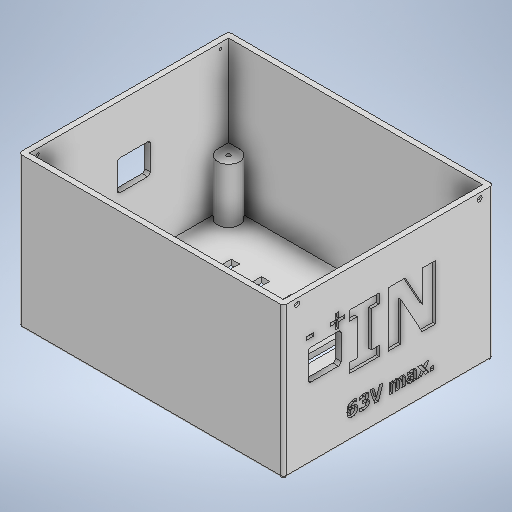
# Autodesk Inventor part: Kondensatorbox
Saved by Autodesk Inventor 2025 (Build 290162010, 162A)
## iProperties
Created: 2024-10-11
Part Number: Kondensatorbox
Material: Generisch
Document SubType Name: Modeling
Designer: max-h
Density: 1 g/cm^3
Appearance: Vorgabe
Author: max-h
Autodesk Inventor part; units mm, degrees
ref_plane "YZ Plane" through (0, 0, 0) normal (1, 0, 0) x (0, 1, 0)
ref_plane "XZ Plane" through (0, 0, 0) normal (0, 1, 0) x (-1, 0, 0)
ref_plane "XY Plane" through (0, 0, 0) normal (0, 0, 1) x (1, 0, 0)
sketch "Skizze1" plane through (0, 0, 0) normal (0, 1, 0) x (-1, 0, 0)
  line L0 (90.5, 0) -> (0, 0) construction
  line L1 (0, 0) -> (0, -70.5) construction
  line L2 (0, -70.5) -> (90.5, -70.5) construction
  line L3 (90.5, -70.5) -> (90.5, 0) construction
  line L4 (93.5, 3) -> (-3, 3)
  line L5 (-3, 3) -> (-3, -73.5)
  line L6 (-3, -73.5) -> (93.5, -73.5)
  line L7 (93.5, -73.5) -> (93.5, 3)
  dimension "d0" = 70.5
  dimension "d1" = 90.5
  dimension "d2" = 3
  dimension "d3" = 3
  dimension "d4" = 3
  dimension "d5" = 3
  constraints: 16 end point, 4 parallel, 2 horizontal, 2 perpendicular, 1 coincident
  measures "d0" distance of L2.end L0.start
  measures "d1" distance of L1.end L2.end
  measures "d2" distance between parallel lines of L7 L3
  measures "d3" distance between parallel lines of L4 L0
  measures "d4" distance between parallel lines of L5 L1
  measures "d5" distance between parallel lines of L6 L2
extrude "Extrusion1" add sketch "Skizze1" along normal blind 55
shell "Wandung1" thickness 2 removed faces 1 at (-29.1667, 55, -22.5)
sketch "Skizze4" plane through (1, 55, -71.5) normal (-1, 0, 0) x (0, 0, 1)
  line L0 (65.5, -29) -> (53.5, -29)
  line L1 (53.5, -29) -> (53.5, -18)
  line L2 (53.5, -18) -> (65.5, -18)
  line L3 (65.5, -18) -> (65.5, -29)
  line L4 (72.5, -53) -> (72.5, 0) projected
  line L5 (72.5, -53) -> (0, -53) projected
  point P0 (71.5, -55)
  dimension "d26" = 7
  dimension "d27" = 12
  dimension "d29" = 11
  dimension "d65" = 24
  constraints: 8 end point, 2 parallel, 1 horizontal, 1 perpendicular
  measures "d26" distance between parallel lines of L4 L3
  measures "d27" distance of L0.start L0.end
  measures "d29" distance of L2.end L0.start
  measures "d65" distance between parallel lines of L5 L0
extrude "Extrusion4" cut sketch "Skizze4" against normal blind 4
sketch "Skizze5" plane through (-91.5, 55, 1) normal (1, 0, 0) x (0, 0, -1)
  line L0 (32, -18) -> (44, -18)
  line L1 (44, -18) -> (44, -29)
  line L2 (44, -29) -> (32, -29)
  line L3 (32, -29) -> (32, -18)
  line L4 (19, -18) -> (19, -29) projected
  line L5 (7, -18) -> (19, -18) projected
  line L6 (0, -53) -> (0, 0) projected
  line L7 (72.5, -53) -> (0, -53) projected
  point P0 (1, -55)
  dimension "d33" = 32
  dimension "d66" = 24
  constraints: 8 end point, 2 equal length, 2 parallel, 1 horizontal, 1 perpendicular
  measures "d33" distance between parallel lines of L6 L3
  measures "d66" distance between parallel lines of L7 L2
extrude "Extrusion5" cut sketch "Skizze5" against normal blind 4
fillet "Rundung1" radius 1 16 edges at (-92.5, 26, -43) (-92.5, 26, -31) (-92.5, 37, -31) (-92.5, 37, -43) (2, 26, -6) (2, 26, -18) (2, 37, -18) (2, 37, -6) (-45.25, 0, 3) (3, 0, -35.25) (-45.25, 0, -73.5) (-93.5, 0, -35.25) (3, 27.5, -73.5) (-93.5, 27.5, -73.5) (3, 27.5, 3) (-93.5, 27.5, 3)
sketch "Skizze6" plane through (3, 0, 3) normal (1, 0, 0) x (0, 0, -1)
  circle A0 centre (5, 53) radius 0.5
  circle A1 centre (71.5, 53) radius 0.5
  line L0 (5, 53) -> (71.5, 53) construction
  line L1 (1, 55) -> (75.5, 55) construction
  line L2 (0, 55) -> (0, 1) projected
  line L3 (76.5, 1) -> (76.5, 55) projected
  point P0 (3, 0)
  dimension "d40" = 2
  dimension "d43" = 1
  dimension "d46" = 5
  dimension "d47" = 5
  constraints: 2 centre point, 2 end point, 1 coincident, 1 equal radius, 1 horizontal
  measures "d40" distance between parallel lines of L1 L0
  measures "d43" diameter of A1
  measures "d46" distance from line of L2 L0.start
  measures "d47" distance from line of L3 A1.centre
extrude "Extrusion6" cut sketch "Skizze6" against normal through all
chamfer "Fasen2" distance 0.4 angle 45 4 edges at (3, 53, -1.5) (3, 53, -68) (-93.5, 53, -68) (-93.5, 53, -1.5)
sketch "Skizze10" plane through (-91.5, 2, -71.5) normal (0, 1, 0) x (1, 0, 0)
  arc A0 (92.5, -68.5) -> (88.5, -72.5) centre (88.5, -68.5) ccw
  line L0 (0, -72.5) -> (92.5, -72.5) projected
  line L1 (92.5, -72.5) -> (92.5, 0) projected
  arc A1 (88.5, 0) -> (92.5, -4) centre (88.5, -4) ccw
  arc A2 (0, -4) -> (4, 0) centre (4, -4) ccw
  arc A3 (4, -72.5) -> (0, -68.5) centre (4, -68.5) ccw
  line L2 (0, 0) -> (0, -72.5) projected
  line L3 (92.5, 0) -> (0, 0) projected
  point P0 (91.5, -71.5)
  dimension "d67" = 4
  dimension "d68" = 4
  dimension "d69" = 4
  dimension "d70" = 4
  dimension "d71" = 4
  dimension "d72" = 4
  dimension "d73" = 4
  dimension "d74" = 4
  dimension "d75" = 8
  constraints: 8 point on circle, 8 point on line, 4 centre point, 3 equal radius
  measures "d67" distance from line of L0 A0.centre
  measures "d68" distance from line of L1 A0.centre
  measures "d69" distance from line of L0 A3.centre
  measures "d70" distance from line of L2 A3.centre
  measures "d71" distance from line of L2 A2.centre
  measures "d72" distance from line of L3 A2.centre
  measures "d73" distance from line of L3 A1.centre
  measures "d74" distance from line of L1 A1.centre
  measures "d75" diameter of A0
extrude "Extrusion10" add sketch "Skizze10" along normal blind 20 contours L1 L0 A0 | A1 L3 L1 | L0 L2 A3 | A2 L2 L3
sketch "Skizze11" plane through (-91.5, 22, -71.5) normal (0, 1, 0) x (1, 0, 0)
  arc A0 (92.5, -68.5) -> (88.5, -72.5) centre (88.5, -68.5) ccw projected
  arc A1 (4, -72.5) -> (0, -68.5) centre (4, -68.5) ccw projected
  line L0 (0, -4) -> (0, 0) projected
  arc A2 (0, -4) -> (4, 0) centre (4, -4) ccw projected
  line L1 (0, 0) -> (4, 0) projected
  arc A3 (88.5, 0) -> (92.5, -4) centre (88.5, -4) ccw projected
  circle A4 centre (88.5, -4) radius 0.75
  circle A5 centre (88.5, -68.5) radius 0.75
  circle A6 centre (4, -68.5) radius 0.75
  circle A7 centre (4, -4) radius 0.75
  point P0 (91.5, -71.5)
  dimension "d78" = 1.5
  constraints: 4 centre point, 4 coincident, 3 equal radius
  measures "d78" diameter of A5
extrude "Extrusion11" cut sketch "Skizze11" against normal blind 10 contours A4 | A5 | A6 | A7
sketch "Skizze12" plane through (-87.5, 2, -71.5) normal (0, 1, 0) x (1, 0, 0)
  line L0 (71.25, -56.25) -> (68.25, -56.25)
  line L1 (68.25, -56.25) -> (68.25, -16.25)
  line L2 (68.25, -16.25) -> (71.25, -16.25)
  line L3 (71.25, -16.25) -> (71.25, -56.25)
  line L4 (60.25, -56.25) -> (57.25, -56.25)
  line L5 (57.25, -56.25) -> (57.25, -16.25)
  line L6 (57.25, -16.25) -> (60.25, -16.25)
  line L7 (60.25, -16.25) -> (60.25, -56.25)
  line L8 (49.25, -56.25) -> (46.25, -56.25)
  line L9 (46.25, -56.25) -> (46.25, -16.25)
  line L10 (46.25, -16.25) -> (49.25, -16.25)
  line L11 (49.25, -16.25) -> (49.25, -56.25)
  line L12 (38.25, -56.25) -> (35.25, -56.25)
  line L13 (35.25, -56.25) -> (35.25, -16.25)
  line L14 (35.25, -16.25) -> (38.25, -16.25)
  line L15 (38.25, -16.25) -> (38.25, -56.25)
  line L16 (27.25, -56.25) -> (24.25, -56.25)
  line L17 (24.25, -56.25) -> (24.25, -16.25)
  line L18 (24.25, -16.25) -> (27.25, -16.25)
  line L19 (27.25, -16.25) -> (27.25, -56.25)
  line L20 (16.25, -56.25) -> (13.25, -56.25)
  line L21 (13.25, -56.25) -> (13.25, -16.25)
  line L22 (13.25, -16.25) -> (16.25, -16.25)
  line L23 (16.25, -16.25) -> (16.25, -56.25)
  line L24 (-4, -4) -> (-4, -68.5) projected
  line L25 (0, -72.5) -> (84.5, -72.5) projected
  point P0 (87.5, -71.5)
  point P1 (57.25, -36.25)
  point P2 (27.25, -36.25)
  point P3 (35.25, -36.25)
  dimension "d81" = 8
  dimension "d82" = 8
  dimension "d83" = 8
  dimension "d84" = 8
  dimension "d85" = 8
  dimension "d86" = 3
  dimension "d87" = 40
  dimension "d88" = 17.25
  dimension "d89" = 16.25
  constraints: 48 end point, 12 parallel, 9 equal length, 6 horizontal, 6 perpendicular, 4 point on line, 3 midpoint, 2 collinear
  measures "d81" distance between parallel lines of L7 L1
  measures "d82" distance from line of L11 point (57.25, -36.25)
  measures "d83" distance between parallel lines of L15 L9
  measures "d84" distance of point (27.25, -36.25) point (35.25, -36.25)
  measures "d85" distance between parallel lines of L23 L17
  measures "d86" distance of L1.end L2.end
  measures "d87" distance of L2.end L0.start
  measures "d88" distance between parallel lines of L24 L21
  measures "d89" distance between parallel lines of L25 L0
extrude "Extrusion12" cut sketch "Skizze12" against normal blind 55
sketch "Skizze13" plane through (3, 1, -72.5) normal (1, 0, 0) x (0, 0, -1)
  line L0 (-52.6804, 40.6521) -> (-18.8731, 40.6521) construction
  line L1 (-18.8731, 40.6521) -> (-18.8731, 5.4097) construction
  line L2 (-18.8731, 5.4097) -> (-52.6804, 5.4097) construction
  line L3 (-52.6804, 5.4097) -> (-52.6804, 40.6521) construction
  line L4 (-40.6545, 20.6521) -> (-51.4162, 20.6521)
  line L5 (-51.4162, 20.6521) -> (-51.4162, 24.1367)
  line L6 (-51.4162, 24.1367) -> (-48.5475, 24.1367)
  line L7 (-48.5475, 24.1367) -> (-48.5475, 37.1675)
  line L8 (-48.5475, 37.1675) -> (-51.4162, 37.1675)
  line L9 (-51.4162, 37.1675) -> (-51.4162, 40.6521)
  line L10 (-51.4162, 40.6521) -> (-40.6545, 40.6521)
  line L11 (-40.6545, 40.6521) -> (-40.6545, 37.1675)
  line L12 (-40.6545, 37.1675) -> (-43.5232, 37.1675)
  line L13 (-43.5232, 37.1675) -> (-43.5232, 24.1367)
  line L14 (-43.5232, 24.1367) -> (-40.6545, 24.1367)
  line L15 (-40.6545, 24.1367) -> (-40.6545, 20.6521)
  line L16 (-20.1844, 20.6521) -> (-25.0143, 20.6521)
  line L17 (-25.0143, 20.6521) -> (-32.729, 34.5905)
  line L18 (-32.729, 34.5905) -> (-32.729, 20.6521)
  line L19 (-32.729, 20.6521) -> (-37.3157, 20.6521)
  line L20 (-37.3157, 20.6521) -> (-37.3157, 40.6521)
  line L21 (-37.3157, 40.6521) -> (-31.1569, 40.6521)
  line L22 (-31.1569, 40.6521) -> (-24.7711, 29.1934)
  line L23 (-24.7711, 29.1934) -> (-24.7711, 40.6521)
  line L24 (-24.7711, 40.6521) -> (-20.1844, 40.6521)
  line L25 (-20.1844, 40.6521) -> (-20.1844, 20.6521)
  spline S0 degree 2 poles (-48.5272, 8.3331) (-48.5272, 7.543) (-49.528, 6.526) (-50.4032, 6.526) knots 0 0 0 1 2 2 2
  spline S1 degree 2 poles (-50.4032, 6.526) (-50.8408, 6.526) (-51.5256, 6.7772) (-51.7647, 7.0243) knots 0 0 0 1 2 2 2
  spline S2 degree 2 poles (-51.7647, 7.0243) (-52.0483, 7.312) (-52.3522, 8.2237) (-52.3522, 8.8598) knots 0 0 0 1 2 2 2
  spline S3 degree 2 poles (-52.3522, 8.8598) (-52.3522, 9.5162) (-52.0686, 10.5373) (-51.7485, 10.9303) knots 0 0 0 1 2 2 2
  spline S4 degree 2 poles (-51.7485, 10.9303) (-51.4446, 11.3031) (-50.4559, 11.7245) (-49.7792, 11.7245) knots 0 0 0 1 2 2 2
  spline S5 degree 2 poles (-49.7792, 11.7245) (-49.5321, 11.7245) (-49.0378, 11.6597) (-48.9486, 11.6394) knots 0 0 0 1 2 2 2
  line L26 (-48.9486, 11.6394) -> (-48.9486, 10.6589)
  line L27 (-48.9486, 10.6589) -> (-49.0378, 10.6589)
  spline S6 degree 2 poles (-49.0378, 10.6589) (-49.1269, 10.7034) (-49.5321, 10.8128) (-49.7914, 10.8128) knots 0 0 0 1 2 2 2
  spline S7 degree 2 poles (-49.7914, 10.8128) (-50.3789, 10.8128) (-51.0191, 10.1929) (-51.0961, 9.6175) knots 0 0 0 1 2 2 2
  spline S8 degree 2 poles (-51.0961, 9.6175) (-50.8489, 9.7755) (-50.3425, 9.9619) (-50.0224, 9.9619) knots 0 0 0 1 2 2 2
  spline S9 degree 2 poles (-50.0224, 9.9619) (-49.7509, 9.9619) (-49.2768, 9.8161) (-49.0945, 9.6783) knots 0 0 0 1 2 2 2
  spline S10 degree 2 poles (-49.0945, 9.6783) (-48.8352, 9.4798) (-48.5272, 8.8355) (-48.5272, 8.3331) knots 0 0 0 1 2 2 2
  spline S11 degree 2 poles (-49.9899, 7.5794) (-49.8927, 7.701) (-49.7874, 7.9846) (-49.7874, 8.2723) knots 0 0 0 1 2 2 2
  spline S12 degree 2 poles (-49.7874, 8.2723) (-49.7874, 8.5154) (-49.9089, 8.8315) (-50.0183, 8.9247) knots 0 0 0 1 2 2 2
  spline S13 degree 2 poles (-50.0183, 8.9247) (-50.1318, 9.0219) (-50.4113, 9.0908) (-50.5694, 9.0908) knots 0 0 0 1 2 2 2
  spline S14 degree 2 poles (-50.5694, 9.0908) (-50.7031, 9.0908) (-50.9786, 9.0219) (-51.1002, 8.9733) knots 0 0 0 1 2 2 2
  spline S15 degree 2 poles (-51.1002, 8.9733) (-51.1002, 8.9409) (-51.1083, 8.7869) (-51.1083, 8.6694) knots 0 0 0 1 2 2 2
  spline S16 degree 2 poles (-51.1083, 8.6694) (-51.1083, 8.2358) (-50.9583, 7.7132) (-50.8408, 7.5794) knots 0 0 0 1 2 2 2
  spline S17 degree 2 poles (-50.8408, 7.5794) (-50.7557, 7.47) (-50.5288, 7.3768) (-50.4073, 7.3768) knots 0 0 0 1 2 2 2
  spline S18 degree 2 poles (-50.4073, 7.3768) (-50.306, 7.3768) (-50.071, 7.4781) (-49.9899, 7.5794) knots 0 0 0 1 2 2 2
  spline S19 degree 2 poles (-44.2444, 8.1467) (-44.2444, 7.778) (-44.5159, 7.1743) (-44.7792, 6.9636) knots 0 0 0 1 2 2 2
  spline S20 degree 2 poles (-44.7792, 6.9636) (-45.0426, 6.7529) (-45.7598, 6.526) (-46.2744, 6.526) knots 0 0 0 1 2 2 2
  spline S21 degree 2 poles (-46.2744, 6.526) (-46.8579, 6.526) (-47.6925, 6.7204) (-47.9559, 6.842) knots 0 0 0 1 2 2 2
  line L28 (-47.9559, 6.842) -> (-47.9559, 7.9279)
  line L29 (-47.9559, 7.9279) -> (-47.8344, 7.9279)
  spline S22 degree 2 poles (-47.8344, 7.9279) (-47.5588, 7.7537) (-46.8173, 7.4944) (-46.5094, 7.4944) knots 0 0 0 1 2 2 2
  spline S23 degree 2 poles (-46.5094, 7.4944) (-46.3271, 7.4944) (-45.9016, 7.5592) (-45.7557, 7.6645) knots 0 0 0 1 2 2 2
  spline S24 degree 2 poles (-45.7557, 7.6645) (-45.6423, 7.7496) (-45.5045, 7.9968) (-45.5045, 8.2196) knots 0 0 0 1 2 2 2
  spline S25 degree 2 poles (-45.5045, 8.2196) (-45.5045, 8.4425) (-45.699, 8.6815) (-45.8611, 8.7383) knots 0 0 0 1 2 2 2
  spline S26 degree 2 poles (-45.8611, 8.7383) (-46.0232, 8.795) (-46.4729, 8.8072) (-46.6472, 8.8072) knots 0 0 0 1 2 2 2
  line L30 (-46.6472, 8.8072) -> (-46.8619, 8.8072)
  line L31 (-46.8619, 8.8072) -> (-46.8619, 9.6864)
  line L32 (-46.8619, 9.6864) -> (-46.6634, 9.6864)
  spline S27 degree 2 poles (-46.6634, 9.6864) (-46.4365, 9.6864) (-46.0515, 9.7269) (-45.9178, 9.7877) knots 0 0 0 1 2 2 2
  spline S28 degree 2 poles (-45.9178, 9.7877) (-45.7841, 9.8525) (-45.6342, 10.0794) (-45.6342, 10.2739) knots 0 0 0 1 2 2 2
  spline S29 degree 2 poles (-45.6342, 10.2739) (-45.6342, 10.4279) (-45.776, 10.6183) (-45.8773, 10.671) knots 0 0 0 1 2 2 2
  spline S30 degree 2 poles (-45.8773, 10.671) (-45.9989, 10.7318) (-46.323, 10.7723) (-46.4365, 10.7723) knots 0 0 0 1 2 2 2
  spline S31 degree 2 poles (-46.4365, 10.7723) (-46.6188, 10.7723) (-47.0037, 10.6872) (-47.182, 10.6183) knots 0 0 0 1 2 2 2
  spline S32 degree 2 poles (-47.182, 10.6183) (-47.3238, 10.5657) (-47.6318, 10.3955) (-47.7047, 10.3509) knots 0 0 0 1 2 2 2
  line L33 (-47.7047, 10.3509) -> (-47.81, 10.3509)
  line L34 (-47.81, 10.3509) -> (-47.81, 11.4206)
  spline S33 degree 2 poles (-47.81, 11.4206) (-47.5507, 11.53) (-46.6755, 11.7367) (-46.2177, 11.7367) knots 0 0 0 1 2 2 2
  spline S34 degree 2 poles (-46.2177, 11.7367) (-45.772, 11.7367) (-45.1156, 11.5827) (-44.8846, 11.4328) knots 0 0 0 1 2 2 2
  spline S35 degree 2 poles (-44.8846, 11.4328) (-44.6293, 11.2747) (-44.3741, 10.7885) (-44.3741, 10.4846) knots 0 0 0 1 2 2 2
  spline S36 degree 2 poles (-44.3741, 10.4846) (-44.3741, 10.0551) (-44.8684, 9.4149) (-45.2736, 9.3217) knots 0 0 0 1 2 2 2
  line L35 (-45.2736, 9.3217) -> (-45.2736, 9.2731)
  spline S37 degree 2 poles (-45.2736, 9.2731) (-45.0953, 9.2488) (-44.7549, 9.1191) (-44.5929, 8.9733) knots 0 0 0 1 2 2 2
  spline S38 degree 2 poles (-44.5929, 8.9733) (-44.4429, 8.8436) (-44.2444, 8.4303) (-44.2444, 8.1467) knots 0 0 0 1 2 2 2
  line L36 (-39.2282, 11.6313) -> (-40.9462, 6.6313)
  line L37 (-40.9462, 6.6313) -> (-42.2549, 6.6313)
  line L38 (-42.2549, 6.6313) -> (-43.9729, 11.6313)
  line L39 (-43.9729, 11.6313) -> (-42.6723, 11.6313)
  line L40 (-42.6723, 11.6313) -> (-41.5823, 8.2399)
  line L41 (-41.5823, 8.2399) -> (-40.4964, 11.6313)
  line L42 (-40.4964, 11.6313) -> (-39.2282, 11.6313)
  line L43 (-32.3157, 6.6313) -> (-32.3157, 8.5154)
  spline S39 degree 2 poles (-32.3157, 8.5154) (-32.3157, 8.795) (-32.336, 9.1759) (-32.3846, 9.2974) knots 0 0 0 1 2 2 2
  spline S40 degree 2 poles (-32.3846, 9.2974) (-32.4373, 9.419) (-32.648, 9.5284) (-32.8384, 9.5284) knots 0 0 0 1 2 2 2
  spline S41 degree 2 poles (-32.8384, 9.5284) (-32.9721, 9.5284) (-33.2314, 9.4109) (-33.3854, 9.3015) knots 0 0 0 1 2 2 2
  line L44 (-33.3854, 9.3015) -> (-33.3854, 6.6313)
  line L45 (-33.3854, 6.6313) -> (-34.5686, 6.6313)
  line L46 (-34.5686, 6.6313) -> (-34.5686, 8.5154)
  spline S42 degree 2 poles (-34.5686, 8.5154) (-34.5686, 8.7909) (-34.5929, 9.1759) (-34.6415, 9.2974) knots 0 0 0 1 2 2 2
  spline S43 degree 2 poles (-34.6415, 9.2974) (-34.6942, 9.419) (-34.9049, 9.5284) (-35.0953, 9.5284) knots 0 0 0 1 2 2 2
  spline S44 degree 2 poles (-35.0953, 9.5284) (-35.2371, 9.5284) (-35.5167, 9.3947) (-35.6463, 9.3015) knots 0 0 0 1 2 2 2
  line L47 (-35.6463, 9.3015) -> (-35.6463, 6.6313)
  line L48 (-35.6463, 6.6313) -> (-36.8214, 6.6313)
  line L49 (-36.8214, 6.6313) -> (-36.8214, 10.4036)
  line L50 (-36.8214, 10.4036) -> (-35.6463, 10.4036)
  line L51 (-35.6463, 10.4036) -> (-35.6463, 9.9862)
  spline S45 degree 2 poles (-35.6463, 9.9862) (-35.3587, 10.2294) (-34.8441, 10.5049) (-34.524, 10.5049) knots 0 0 0 1 2 2 2
  spline S46 degree 2 poles (-34.524, 10.5049) (-34.1796, 10.5049) (-33.6528, 10.1767) (-33.5151, 9.8485) knots 0 0 0 1 2 2 2
  spline S47 degree 2 poles (-33.5151, 9.8485) (-33.1788, 10.1645) (-32.5791, 10.5049) (-32.2711, 10.5049) knots 0 0 0 1 2 2 2
  spline S48 degree 2 poles (-32.2711, 10.5049) (-32.0078, 10.5049) (-31.5904, 10.3388) (-31.4486, 10.1686) knots 0 0 0 1 2 2 2
  spline S49 degree 2 poles (-31.4486, 10.1686) (-31.2906, 9.9862) (-31.1326, 9.4879) (-31.1326, 9.0867) knots 0 0 0 1 2 2 2
  line L52 (-31.1326, 9.0867) -> (-31.1326, 6.6313)
  line L53 (-31.1326, 6.6313) -> (-32.3157, 6.6313)
  spline S50 degree 2 poles (-28.1828, 7.0324) (-28.3044, 6.9311) (-28.4948, 6.7691) (-28.6569, 6.688) knots 0 0 0 1 2 2 2
  spline S51 degree 2 poles (-28.6569, 6.688) (-28.8149, 6.611) (-29.1147, 6.53) (-29.3822, 6.53) knots 0 0 0 1 2 2 2
  spline S52 degree 2 poles (-29.3822, 6.53) (-29.8846, 6.53) (-30.5451, 7.2026) (-30.5451, 7.7132) knots 0 0 0 1 2 2 2
  spline S53 degree 2 poles (-30.5451, 7.7132) (-30.5451, 8.1305) (-30.2087, 8.6491) (-29.8927, 8.7991) knots 0 0 0 1 2 2 2
  spline S54 degree 2 poles (-29.8927, 8.7991) (-29.5726, 8.953) (-28.6852, 9.0746) (-28.1747, 9.107) knots 0 0 0 1 2 2 2
  line L54 (-28.1747, 9.107) -> (-28.1747, 9.1273)
  spline S55 degree 2 poles (-28.1747, 9.1273) (-28.1747, 9.4392) (-28.6366, 9.6783) (-29.0985, 9.6783) knots 0 0 0 1 2 2 2
  spline S56 degree 2 poles (-29.0985, 9.6783) (-29.3052, 9.6783) (-29.8643, 9.5284) (-30.1277, 9.4109) knots 0 0 0 1 2 2 2
  line L55 (-30.1277, 9.4109) -> (-30.229, 9.4109)
  line L56 (-30.229, 9.4109) -> (-30.229, 10.3226)
  spline S57 degree 2 poles (-30.229, 10.3226) (-30.0548, 10.3712) (-29.2768, 10.5089) (-28.8797, 10.5089) knots 0 0 0 1 2 2 2
  spline S58 degree 2 poles (-28.8797, 10.5089) (-27.9073, 10.5089) (-27.0159, 9.8606) (-27.0159, 9.1961) knots 0 0 0 1 2 2 2
  line L57 (-27.0159, 9.1961) -> (-27.0159, 6.6313)
  line L58 (-27.0159, 6.6313) -> (-28.1828, 6.6313)
  line L59 (-28.1828, 6.6313) -> (-28.1828, 7.0324)
  line L60 (-28.1828, 7.6159) -> (-28.1828, 8.3979)
  spline S59 degree 2 poles (-28.1828, 8.3979) (-28.4827, 8.3696) (-28.8514, 8.325) (-29.0297, 8.2602) knots 0 0 0 1 2 2 2
  spline S60 degree 2 poles (-29.0297, 8.2602) (-29.1877, 8.2075) (-29.3579, 7.9887) (-29.3579, 7.8104) knots 0 0 0 1 2 2 2
  spline S61 degree 2 poles (-29.3579, 7.8104) (-29.3579, 7.547) (-29.0702, 7.3485) (-28.7906, 7.3485) knots 0 0 0 1 2 2 2
  spline S62 degree 2 poles (-28.7906, 7.3485) (-28.6366, 7.3485) (-28.3125, 7.4903) (-28.1828, 7.6159) knots 0 0 0 1 2 2 2
  line L61 (-22.4251, 6.6313) -> (-23.8027, 6.6313)
  line L62 (-23.8027, 6.6313) -> (-24.5199, 7.7132)
  line L63 (-24.5199, 7.7132) -> (-25.2574, 6.6313)
  line L64 (-25.2574, 6.6313) -> (-26.6066, 6.6313)
  line L65 (-26.6066, 6.6313) -> (-25.2168, 8.5195)
  line L66 (-25.2168, 8.5195) -> (-26.5823, 10.4036)
  line L67 (-26.5823, 10.4036) -> (-25.2047, 10.4036)
  line L68 (-25.2047, 10.4036) -> (-24.4997, 9.342)
  line L69 (-24.4997, 9.342) -> (-23.7906, 10.4036)
  line L70 (-23.7906, 10.4036) -> (-22.4413, 10.4036)
  line L71 (-22.4413, 10.4036) -> (-23.8068, 8.5478)
  line L72 (-23.8068, 8.5478) -> (-22.4251, 6.6313)
  line L73 (-20.772, 6.6313) -> (-21.9592, 6.6313)
  line L74 (-21.9592, 6.6313) -> (-21.9592, 7.9522)
  line L75 (-21.9592, 7.9522) -> (-20.772, 7.9522)
  line L76 (-20.772, 7.9522) -> (-20.772, 6.6313)
  point P0 (-72.5, -1)
  constraints: 2 other
extrude "Extrusion13" cut sketch "Skizze13" against normal blind 1
sketch "Skizze14" plane through (-93.5, 1, -72.5) normal (-1, 0, 0) x (0, 0, 1)
  line L0 (14.2808, 23.4416) -> (59.1282, 23.4416) construction
  line L1 (59.1282, 23.4416) -> (59.1282, 6.984) construction
  line L2 (59.1282, 6.984) -> (14.2808, 6.984) construction
  line L3 (14.2808, 6.984) -> (14.2808, 23.4416) construction
  spline S0 degree 2 poles (29.4875, 15.6255) (29.4875, 11.9788) (25.5977, 7.8095) (22.2184, 7.8095) knots 0 0 0 1 2 2 2
  spline S1 degree 2 poles (22.2184, 7.8095) (18.827, 7.8095) (14.9615, 12.0275) (14.9615, 15.6255) knots 0 0 0 1 2 2 2
  spline S2 degree 2 poles (14.9615, 15.6255) (14.9615, 19.2357) (18.827, 23.4416) (22.2184, 23.4416) knots 0 0 0 1 2 2 2
  spline S3 degree 2 poles (22.2184, 23.4416) (25.5977, 23.4416) (29.4875, 19.26) (29.4875, 15.6255) knots 0 0 0 1 2 2 2
  spline S4 degree 2 poles (25.5977, 15.6255) (25.5977, 16.9748) (25.0507, 18.8589) (24.5766, 19.4545) knots 0 0 0 1 2 2 2
  spline S5 degree 2 poles (24.5766, 19.4545) (24.1025, 20.0745) (22.887, 20.6093) (22.2306, 20.6093) knots 0 0 0 1 2 2 2
  spline S6 degree 2 poles (22.2306, 20.6093) (21.5377, 20.6093) (20.4072, 20.1109) (19.8845, 19.4788) knots 0 0 0 1 2 2 2
  spline S7 degree 2 poles (19.8845, 19.4788) (19.4226, 18.8954) (18.8513, 16.9626) (18.8513, 15.6255) knots 0 0 0 1 2 2 2
  spline S8 degree 2 poles (18.8513, 15.6255) (18.8513, 14.2398) (19.3983, 12.4164) (19.8724, 11.7965) knots 0 0 0 1 2 2 2
  spline S9 degree 2 poles (19.8724, 11.7965) (20.3464, 11.1766) (21.5742, 10.6417) (22.2306, 10.6417) knots 0 0 0 1 2 2 2
  spline S10 degree 2 poles (22.2306, 10.6417) (22.8991, 10.6417) (24.139, 11.213) (24.5887, 11.8208) knots 0 0 0 1 2 2 2
  spline S11 degree 2 poles (24.5887, 11.8208) (25.075, 12.4772) (25.5977, 14.2155) (25.5977, 15.6255) knots 0 0 0 1 2 2 2
  spline S12 degree 2 poles (37.7897, 7.8095) (34.763, 7.8095) (31.5053, 10.7268) (31.5053, 13.5469) knots 0 0 0 1 2 2 2
  line L4 (31.5053, 13.5469) -> (31.5053, 23.1255)
  line L5 (31.5053, 23.1255) -> (35.2735, 23.1255)
  line L6 (35.2735, 23.1255) -> (35.2735, 13.7657)
  spline S13 degree 2 poles (35.2735, 13.7657) (35.2735, 12.1976) (36.4526, 10.666) (37.7897, 10.666) knots 0 0 0 1 2 2 2
  spline S14 degree 2 poles (37.7897, 10.666) (39.0904, 10.666) (40.3059, 12.1369) (40.3059, 13.7657) knots 0 0 0 1 2 2 2
  line L7 (40.3059, 13.7657) -> (40.3059, 23.1255)
  line L8 (40.3059, 23.1255) -> (44.0742, 23.1255)
  line L9 (44.0742, 23.1255) -> (44.0742, 13.5591)
  spline S15 degree 2 poles (44.0742, 13.5591) (44.0742, 10.7876) (40.9016, 7.8095) (37.7897, 7.8095) knots 0 0 0 1 2 2 2
  line L10 (49.8481, 8.1255) -> (49.8481, 20.2689)
  line L11 (49.8481, 20.2689) -> (45.4113, 20.2689)
  line L12 (45.4113, 20.2689) -> (45.4113, 23.1255)
  line L13 (45.4113, 23.1255) -> (58.0531, 23.1255)
  line L14 (58.0531, 23.1255) -> (58.0531, 20.2689)
  line L15 (58.0531, 20.2689) -> (53.6163, 20.2689)
  line L16 (53.6163, 20.2689) -> (53.6163, 8.1255)
  line L17 (53.6163, 8.1255) -> (49.8481, 8.1255)
  point P0 (72.5, -1)
  constraints: 2 other
extrude "Extrusion14" cut sketch "Skizze14" against normal blind 1
sketch "Skizze15" plane through (3, 1, -72.5) normal (1, 0, 0) x (0, 0, -1)
  line L0 (-67.6161, 42.1067) -> (-53.353, 42.1067) construction
  line L1 (-53.353, 42.1067) -> (-53.353, 38.1805) construction
  line L2 (-53.353, 38.1805) -> (-67.6161, 38.1805) construction
  line L3 (-67.6161, 38.1805) -> (-67.6161, 42.1067) construction
  line L4 (-64.5043, 38.9852) -> (-67.1737, 38.9852)
  line L5 (-67.1737, 38.9852) -> (-67.1737, 40.1035)
  line L6 (-67.1737, 40.1035) -> (-64.5043, 40.1035)
  line L7 (-64.5043, 40.1035) -> (-64.5043, 38.9852)
  line L8 (-53.2531, 39.0192) -> (-55.3147, 39.0192)
  line L9 (-55.3147, 39.0192) -> (-55.3147, 36.9722)
  line L10 (-55.3147, 36.9722) -> (-56.3795, 36.9722)
  line L11 (-56.3795, 36.9722) -> (-56.3795, 39.0192)
  line L12 (-56.3795, 39.0192) -> (-58.4411, 39.0192)
  line L13 (-58.4411, 39.0192) -> (-58.4411, 40.0597)
  line L14 (-58.4411, 40.0597) -> (-56.3795, 40.0597)
  line L15 (-56.3795, 40.0597) -> (-56.3795, 42.1067)
  line L16 (-56.3795, 42.1067) -> (-55.3147, 42.1067)
  line L17 (-55.3147, 42.1067) -> (-55.3147, 40.0597)
  line L18 (-55.3147, 40.0597) -> (-53.2531, 40.0597)
  line L19 (-53.2531, 40.0597) -> (-53.2531, 39.0192)
  point P0 (-72.5, -1)
  constraints: 2 other
extrude "Extrusion15" cut sketch "Skizze15" against normal blind 1
